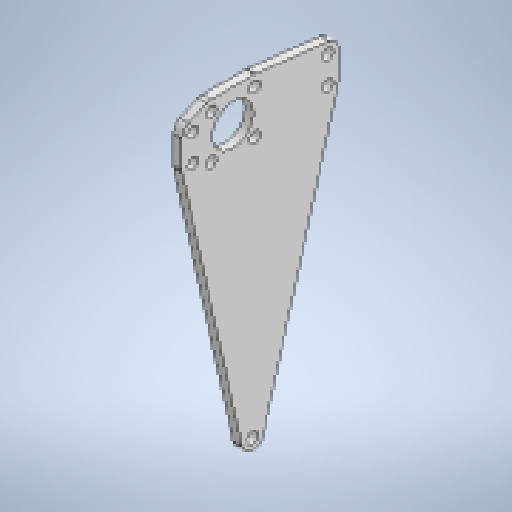
# Autodesk Inventor part: IntakeSlidePlate1.0
Saved by Autodesk Inventor 2023 (Build 270158000, 158)
## iProperties
Created: 2022-10-12
Part Number: IntakeSlidePlate1.0
Material: Generic
Document SubType Name: Modeling
Designer: deli
Density: 1 g/cm^3
Appearance: Default
Author: deli
Autodesk Inventor part; units mm, degrees
ref_plane "YZ Plane" through (0, 0, 0) normal (1, 0, 0) x (0, 1, 0)
ref_plane "XZ Plane" through (0, 0, 0) normal (0, 1, 0) x (-1, 0, 0)
ref_plane "XY Plane" through (0, 0, 0) normal (0, 0, 1) x (1, 0, 0)
sketch "Sketch1" plane through (0, 0, 0) normal (1, 0, 0) x (0, 1, 0)
  circle A0 centre (-130.5395, -37.2207) radius 2
  arc A1 (-131.4148, -33.3176) -> (-131.6229, -41.0712) centre (-130.5395, -37.2207) ccw
  line L0 (-33.3148, -11.3176) -> (-131.4148, -33.3176)
  line L1 (-33.5229, -68.6712) -> (-131.6229, -41.0712)
  line L2 (-32.4395, -11.2207) -> (-22.4395, -11.2207)
  line L3 (-32.4395, -68.8207) -> (-22.4395, -68.8207)
  circle A2 centre (-27.4395, -30.0207) radius 7.5
  circle A3 centre (-32.4395, -15.2207) radius 2
  circle A4 centre (-22.4395, -15.2207) radius 2
  arc A5 (-18.7799, -13.6061) -> (-22.4395, -11.2207) centre (-22.4395, -15.2207) ccw
  circle A6 centre (-22.4395, -64.8207) radius 2
  circle A7 centre (-32.4395, -64.8207) radius 2
  arc A8 (-33.5229, -68.6712) -> (-32.4395, -68.8207) centre (-32.4395, -64.8207) ccw
  arc A9 (-22.4395, -68.8207) -> (-18.4644, -65.2657) centre (-22.4395, -64.8207) ccw
  arc A10 (-32.4395, -11.2207) -> (-33.3148, -11.3176) centre (-32.4395, -15.2207) ccw
  line L4 (-43.9395, -13.7003) -> (-43.9395, -65.7405) construction
  line L5 (-52.9395, -15.7187) -> (-52.9395, -63.2084) construction
  circle A11 centre (-19.4395, -22.0207) radius 2
  circle A12 centre (-19.4395, -38.0207) radius 2
  circle A13 centre (-35.4395, -22.0207) radius 2
  circle A14 centre (-35.4395, -38.0207) radius 2
  line L6 (-19.4395, -22.0207) -> (-19.4395, -38.0207) construction
  line L7 (-19.4395, -38.0207) -> (-35.4395, -38.0207) construction
  line L8 (-35.4395, -38.0207) -> (-35.4395, -22.0207) construction
  line L9 (-35.4395, -22.0207) -> (-19.4395, -22.0207) construction
  circle A15 centre (-27.4395, -30.0207) radius 9.3137 construction
  line L10 (-15.4395, -22.0207) -> (-15.4395, -38.0207)
  line L11 (-15.7799, -20.4061) -> (-18.7799, -13.6061)
  arc A16 (-15.4395, -22.0207) -> (-15.7799, -20.4061) centre (-19.4395, -22.0207) ccw
  line L12 (-15.4644, -38.4657) -> (-18.4644, -65.2657)
  arc A17 (-15.4644, -38.4657) -> (-15.4395, -38.0207) centre (-19.4395, -38.0207) ccw
  point P0 (0, 0)
  dimension "d2" = 4
  dimension "d5" = 8
  dimension "d11" = 26
  dimension "d12" = 15
  dimension "d14" = 4
  dimension "d15" = 14.8
  dimension "d16" = 10
  dimension "d17" = 4
  dimension "d18" = 5
  dimension "d19" = 10
  dimension "d20" = 49.6
  dimension "d21" = 49.6
  dimension "d23" = 9
  dimension "d25" = 77.6
  dimension "d29" = 16
  dimension "d31" = 0
  dimension "d32" = 11.5
  dimension "d33" = 28.5
  constraints: 26 end point, 18 centre point, 16 tangent, 14 point on circle, 12 equal radius, 8 coincident, 4 perpendicular, 4 point on line, 3 horizontal, 1 parallel, 1 vertical
  measures "d2" diameter of A0
  measures "d5" diameter of A1
  measures "d11" distance from line of A0.centre L2
  measures "d12" diameter of A2
  measures "d14" distance from line of L2 A3.centre
  measures "d15" vertical distance of A2.centre A3.centre
  measures "d16" distance of A3.centre A4.centre
  measures "d17" distance from line of L2 A4.centre
  measures "d18" horizontal distance of A2.centre A3.centre
  measures "d19" distance of A7.centre A6.centre
  measures "d20" distance of A6.centre A4.centre
  measures "d21" distance of A7.centre A3.centre
  measures "d23" distance between parallel lines of L4 L5
  measures "d25" distance from line of A0.centre L5
  measures "d29" distance of L6.start L6.end
  measures "d31" horizontal distance of A6.centre A4.centre
  measures "d32" distance from line of A3.centre L4
  measures "d33" distance between parallel lines of L4 L10
extrude "Extrusion1" add sketch "Sketch1" along normal blind 3.175
equation "\"d17\" = d14"
equation "\"d18\" = 0.5 * d16"
equation "\"d19\" = d16"
equation "\"d21\" = d20"
body "Solid1"
